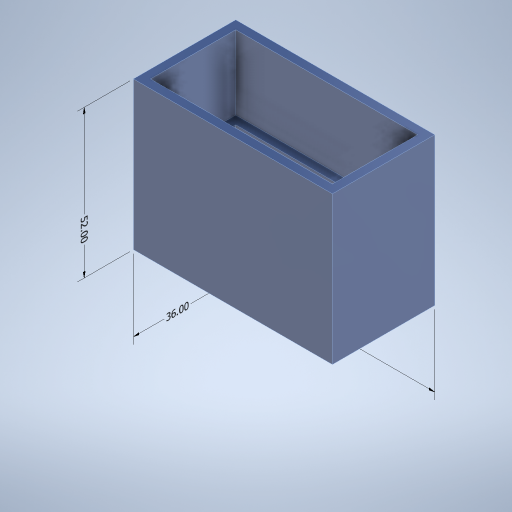
# Autodesk Inventor part: Capsula
Saved by Autodesk Inventor 2023 (Build 270158000, 158)
## iProperties
Created: 2023-03-19
Part Number: Capsula
Material: Plástico PET
Document SubType Name: Modeling
Designer: sergi
Density: 1.541 g/cm^3
Appearance: Satinado con motas - Azul
Author: sergi
Autodesk Inventor part; units mm, degrees
ref_plane "YZ Plane" through (0, 0, 0) normal (1, 0, 0) x (0, 1, 0)
ref_plane "XZ Plane" through (0, 0, 0) normal (0, 1, 0) x (-1, 0, 0)
ref_plane "XY Plane" through (0, 0, 0) normal (0, 0, 1) x (1, 0, 0)
sketch "Boceto1" plane through (0, 0, 0) normal (0, 1, 0) x (-1, 0, 0)
  line L0 (-35, 18) -> (35, 18)
  line L1 (35, 18) -> (35, -18)
  line L2 (35, -18) -> (-35, -18)
  line L3 (-35, -18) -> (-35, 18)
  line L4 (-35, 18) -> (35, -18) construction
  line L5 (35, 18) -> (-35, -18) construction
  line L6 (-32, 15) -> (32, 15)
  line L7 (32, 15) -> (32, -15)
  line L8 (32, -15) -> (-32, -15)
  line L9 (-32, -15) -> (-32, 15)
  line L10 (-32, 15) -> (32, -15) construction
  line L11 (32, 15) -> (-32, -15) construction
  point P0 (0, 0)
  dimension "d0" = 70
  dimension "d1" = 36
  dimension "d2" = 3
  dimension "d3" = 3
  constraints: 24 end point, 4 midpoint, 4 parallel, 2 horizontal, 2 perpendicular
  measures "d0" distance of L1.end L2.end
  measures "d1" distance of L0.end L1.end
  measures "d2" distance between parallel lines of L1 L7
  measures "d3" distance between parallel lines of L2 L8
extrude "Extrusión1" add sketch "Boceto1" along normal blind 3 contours L6 L7 L8 L9
extrude "Extrusión2" add sketch "Boceto1" along normal blind 23
sketch "Boceto2" plane through (0, 23, 0) normal (0, 1, 0) x (1, 0, 0)
  line L0 (35, 18) -> (-35, 18) projected
  line L1 (35, -18) -> (-35, -18)
  line L2 (-35, -18) -> (-35, 18)
  line L3 (-35, 18) -> (35, 18)
  line L4 (35, 18) -> (35, -18)
  line L5 (35, -18) -> (-35, 18) construction
  line L6 (-35, -18) -> (35, 18) construction
  line L7 (29, -12) -> (-29, -12)
  line L8 (-29, -12) -> (-29, 12)
  line L9 (-29, 12) -> (29, 12)
  line L10 (29, 12) -> (29, -12)
  line L11 (29, -12) -> (-29, 12) construction
  line L12 (-29, -12) -> (29, 12) construction
  point P0 (0, 0)
  dimension "d8" = 6
  dimension "d9" = 6
  constraints: 24 end point, 4 midpoint, 4 parallel, 2 horizontal, 2 perpendicular
  measures "d8" distance between parallel lines of L2 L8
  measures "d9" distance between parallel lines of L0 L9
extrude "Extrusión3" add sketch "Boceto2" along normal blind 3
sketch "Boceto3" plane through (0, 26, 0) normal (0, 1, 0) x (1, 0, 0)
  point P0 (0, 0)
sketch "Boceto4" plane through (0, 26, 0) normal (0, 1, 0) x (1, 0, 0)
  line L0 (-35, 18) -> (-35, -18) projected
  line L1 (35, -18) -> (-35, -18)
  line L2 (-35, -18) -> (-35, 18)
  line L3 (-35, 18) -> (35, 18)
  line L4 (35, 18) -> (35, -18)
  line L5 (35, -18) -> (-35, 18) construction
  line L6 (-35, -18) -> (35, 18) construction
  line L7 (32, -15) -> (-32, -15)
  line L8 (-32, -15) -> (-32, 15)
  line L9 (-32, 15) -> (32, 15)
  line L10 (32, 15) -> (32, -15)
  line L11 (32, -15) -> (-32, 15) construction
  line L12 (-32, -15) -> (32, 15) construction
  point P0 (0, 0)
  dimension "d21" = 3
  dimension "d22" = 3
  constraints: 24 end point, 4 midpoint, 4 parallel, 2 horizontal, 2 perpendicular
  measures "d21" distance between parallel lines of L0 L8
  measures "d22" distance between parallel lines of L3 L9
extrude "Extrusión4" add sketch "Boceto4" along normal blind 26
